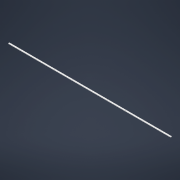
# Autodesk Inventor part: SP28V1 Seguro Acrilico
Saved by Autodesk Inventor 2021.2 (Build 252289000, 289)
## iProperties
Created: 2026-07-28
Part Number: SP28V1 Seguro Acrilico
Material: Steel, Carbon
Document SubType Name: Modeling
Designer: nelso
Density: 7.87 g/cm^3
Appearance: White
Mass: 507.558 g
Surface Area: 522.955 cm^2
Volume: 64.4928 cm^3
Author: nelso
Autodesk Inventor part; units mm, degrees
ref_plane "YZ Plane" through (0, 0, 0) normal (1, 0, 0) x (0, 1, 0)
ref_plane "XZ Plane" through (0, 0, 0) normal (0, 1, 0) x (-1, 0, 0)
ref_plane "XY Plane" through (0, 0, 0) normal (0, 0, 1) x (1, 0, 0)
sketch "Sketch1" plane through (0, 0, 0) normal (0, 1, 0) x (-1, 0, 0)
  line L0 (-825, 6.35) -> (825, 6.35)
  line L1 (825, 6.35) -> (825, -6.35)
  line L2 (825, -6.35) -> (-825, -6.35)
  line L3 (-825, -6.35) -> (-825, 6.35)
  line L4 (-825, 6.35) -> (825, -6.35) construction
  line L5 (825, 6.35) -> (-825, -6.35) construction
  point P0 (0, 0)
  dimension "d0" = 1650
  dimension "d1" = 12.7
  constraints: 12 end point, 2 midpoint, 2 parallel, 1 horizontal, 1 perpendicular
  measures "d0" distance of L1.end L2.end
  measures "d1" distance of L0.end L1.end
extrude "Extrusion1" add sketch "Sketch1" along normal blind 3.1
sketch "Sketch2" plane through (0, 3.1, 0) normal (0, 1, 0) x (1, 0, 0)
  circle A0 centre (0, 0) radius 2.25
  dimension "d4" = 4.5
  constraints: 1 centre point, 1 coincident
  measures "d4" diameter of A0
extrude "Extrusion2" cut sketch "Sketch2" against normal blind 3.1
sketch "Sketch4" plane through (0, 3.1, 0) normal (0, 1, 0) x (1, 0, 0)
  line L0 (-825, -6.35) -> (825, -6.35) projected
  line L1 (825, 6.35) -> (-825, 6.35) projected
  line L2 (-825, -6.35) -> (825, -6.35)
  line L3 (825, -6.35) -> (825, 6.35)
  line L4 (825, 6.35) -> (-825, 6.35)
  line L5 (-825, 6.35) -> (-825, -6.35)
  circle A0 centre (0, 0) radius 2.25
  circle A1 centre (180, 0) radius 2.25
  circle A2 centre (360, 0) radius 2.25
  circle A3 centre (540, 0) radius 2.25
  circle A4 centre (720, 0) radius 2.25
  circle A5 centre (-180, 0) radius 2.25
  circle A6 centre (0, 0) radius 2.25
  circle A7 centre (180, 0) radius 2.25
  circle A8 centre (360, 0) radius 2.25
  circle A9 centre (540, 0) radius 2.25
  circle A10 centre (-360, 0) radius 2.25
  circle A11 centre (-180, 0) radius 2.25
  circle A12 centre (0, 0) radius 2.25
  circle A13 centre (180, 0) radius 2.25
  circle A14 centre (360, 0) radius 2.25
  circle A15 centre (-540, 0) radius 2.25
  circle A16 centre (-360, 0) radius 2.25
  circle A17 centre (-180, 0) radius 2.25
  circle A18 centre (0, 0) radius 2.25
  circle A19 centre (180, 0) radius 2.25
  circle A20 centre (-720, 0) radius 2.25
  circle A21 centre (-540, 0) radius 2.25
  circle A22 centre (-360, 0) radius 2.25
  circle A23 centre (-180, 0) radius 2.25
  circle A24 centre (0, 0) radius 2.25
  dimension "d9" = 180
  dimension "d12" = 180
  constraints: 25 centre point, 8 end point, 3 horizontal, 2 parallel, 1 coincident, 1 perpendicular, 48 other
  measures "d9" distance of A0.centre A1.centre
  measures "d12" distance of A0.centre A5.centre
extrude "Extrusion3" cut sketch "Sketch4" against normal blind 180 contours A0 | A1 | A2 | A3 | A4 | A5 | A10 | A15 | A20
fillet "Fillet1" radius 3 4 edges at (825, 1.55, 6.35) (825, 1.55, -6.35) (-825, 1.55, -6.35) (-825, 1.55, 6.35)
equation "\"d15\" = d9"
body "Solid1"
